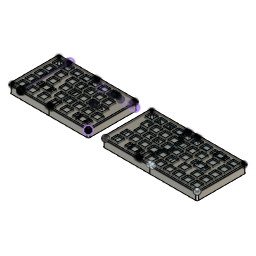
gKeyboard (Autodesk Fusion 360 design; units mm, degrees)
Autodesk Fusion 360 part; units mm, degrees
(part 1 of 3)
sketch "스케치2" plane through (0, 0, 0) normal (0, 0, 1) x (1, 0, 0) in component "leftKey"
  line L0 (0, 0) -> (-142.1125, 0)
  line L1 (-142.1125, 0) -> (-142.1125, 103.25)
  line L2 (-142.1125, 103.25) -> (0, 103.25)
  line L3 (0, 103.25) -> (0, 0)
  circle A0 centre (-3.1, 3.1) radius 1.55
  circle A1 centre (-139.0125, 3.1) radius 1.55
  line L4 (-137.2063, 20.525) -> (-123.2063, 20.525)
  line L5 (-123.2063, 20.525) -> (-123.2063, 6.525)
  line L6 (-123.2063, 6.525) -> (-137.2063, 6.525)
  line L7 (-137.2063, 6.525) -> (-137.2063, 20.525)
  line L8 (-99.3938, 6.525) -> (-113.3938, 6.525)
  line L9 (-113.3938, 6.525) -> (-113.3938, 20.525)
  line L10 (-113.3938, 20.525) -> (-99.3938, 20.525)
  line L11 (-99.3938, 20.525) -> (-99.3938, 6.525)
  line L12 (-75.5813, 6.525) -> (-89.5813, 6.525)
  line L13 (-89.5813, 6.525) -> (-89.5813, 20.525)
  line L14 (-89.5813, 20.525) -> (-75.5813, 20.525)
  line L15 (-75.5813, 20.525) -> (-75.5813, 6.525)
  line L16 (-51.7688, 6.525) -> (-65.7688, 6.525)
  line L17 (-65.7688, 6.525) -> (-65.7688, 20.525)
  line L18 (-65.7688, 20.525) -> (-51.7688, 20.525)
  line L19 (-51.7688, 20.525) -> (-51.7688, 6.525)
  line L20 (-82.725, 25.575) -> (-96.725, 25.575)
  line L21 (-96.725, 39.575) -> (-82.725, 39.575)
  line L22 (-96.725, 25.575) -> (-96.725, 39.575)
  line L23 (-82.725, 39.575) -> (-82.725, 25.575)
  line L24 (-63.675, 25.575) -> (-77.675, 25.575)
  line L25 (-77.675, 25.575) -> (-77.675, 39.575)
  line L26 (-63.675, 39.575) -> (-63.675, 25.575)
  line L27 (-77.675, 39.575) -> (-63.675, 39.575)
  line L28 (-44.625, 25.575) -> (-58.625, 25.575)
  line L29 (-58.625, 25.575) -> (-58.625, 39.575)
  line L30 (-44.625, 39.575) -> (-44.625, 25.575)
  line L31 (-58.625, 39.575) -> (-44.625, 39.575)
  line L32 (-25.575, 25.575) -> (-39.575, 25.575)
  line L33 (-39.575, 25.575) -> (-39.575, 39.575)
  line L34 (-25.575, 39.575) -> (-25.575, 25.575)
  line L35 (-39.575, 39.575) -> (-25.575, 39.575)
  line L36 (-6.525, 25.575) -> (-20.525, 25.575)
  line L37 (-20.525, 25.575) -> (-20.525, 39.575)
  line L38 (-6.525, 39.575) -> (-6.525, 25.575)
  line L39 (-20.525, 39.575) -> (-6.525, 39.575)
  line L40 (-132.4438, 58.625) -> (-118.4438, 58.625)
  line L41 (-132.4438, 44.625) -> (-132.4438, 58.625)
  line L42 (-118.4438, 58.625) -> (-118.4438, 44.625)
  line L43 (-118.4438, 44.625) -> (-132.4438, 44.625)
  line L44 (-106.25, 58.625) -> (-92.25, 58.625)
  line L45 (-106.25, 44.625) -> (-106.25, 58.625)
  line L46 (-92.25, 58.625) -> (-92.25, 44.625)
  line L47 (-92.25, 44.625) -> (-106.25, 44.625)
  line L48 (-73.2, 44.625) -> (-87.2, 44.625)
  line L49 (-87.2, 44.625) -> (-87.2, 58.625)
  line L50 (-73.2, 58.625) -> (-73.2, 44.625)
  line L51 (-87.2, 58.625) -> (-73.2, 58.625)
  line L52 (-54.15, 44.625) -> (-68.15, 44.625)
  line L53 (-68.15, 44.625) -> (-68.15, 58.625)
  line L54 (-54.15, 58.625) -> (-54.15, 44.625)
  line L55 (-68.15, 58.625) -> (-54.15, 58.625)
  line L56 (-35.1, 44.625) -> (-49.1, 44.625)
  line L57 (-49.1, 44.625) -> (-49.1, 58.625)
  line L58 (-35.1, 58.625) -> (-35.1, 44.625)
  line L59 (-49.1, 58.625) -> (-35.1, 58.625)
  line L60 (-16.05, 44.625) -> (-30.05, 44.625)
  line L61 (-30.05, 44.625) -> (-30.05, 58.625)
  line L62 (-16.05, 58.625) -> (-16.05, 44.625)
  line L63 (-30.05, 58.625) -> (-16.05, 58.625)
  line L64 (-120.825, 63.675) -> (-134.825, 63.675)
  line L65 (-134.825, 63.675) -> (-134.825, 77.675)
  line L66 (-120.825, 77.675) -> (-120.825, 63.675)
  line L67 (-134.825, 77.675) -> (-120.825, 77.675)
  line L68 (-111.0125, 63.675) -> (-111.0125, 77.675)
  line L69 (-97.0125, 63.675) -> (-111.0125, 63.675)
  line L70 (-97.0125, 77.675) -> (-97.0125, 63.675)
  line L71 (-111.0125, 77.675) -> (-97.0125, 77.675)
  line L72 (-91.9625, 77.675) -> (-77.9625, 77.675)
  line L73 (-77.9625, 77.675) -> (-77.9625, 63.675)
  line L74 (-77.9625, 63.675) -> (-91.9625, 63.675)
  line L75 (-91.9625, 63.675) -> (-91.9625, 77.675)
  line L76 (-72.9125, 77.675) -> (-58.9125, 77.675)
  line L77 (-58.9125, 77.675) -> (-58.9125, 63.675)
  line L78 (-58.9125, 63.675) -> (-72.9125, 63.675)
  line L79 (-72.9125, 63.675) -> (-72.9125, 77.675)
  line L80 (-53.8625, 77.675) -> (-39.8625, 77.675)
  line L81 (-39.8625, 77.675) -> (-39.8625, 63.675)
  line L82 (-39.8625, 63.675) -> (-53.8625, 63.675)
  line L83 (-53.8625, 63.675) -> (-53.8625, 77.675)
  line L84 (-34.8125, 77.675) -> (-20.8125, 77.675)
  line L85 (-20.8125, 77.675) -> (-20.8125, 63.675)
  line L86 (-20.8125, 63.675) -> (-34.8125, 63.675)
  line L87 (-34.8125, 63.675) -> (-34.8125, 77.675)
  line L88 (-125.5875, 82.725) -> (-139.5875, 82.725)
  line L89 (-139.5875, 82.725) -> (-139.5875, 96.725)
  line L90 (-125.5875, 96.725) -> (-125.5875, 82.725)
  line L91 (-139.5875, 96.725) -> (-125.5875, 96.725)
  line L92 (-106.5375, 96.725) -> (-106.5375, 82.725)
  line L93 (-106.5375, 82.725) -> (-120.5375, 82.725)
  line L94 (-120.5375, 82.725) -> (-120.5375, 96.725)
  line L95 (-120.5375, 96.725) -> (-106.5375, 96.725)
  line L96 (-87.4875, 96.725) -> (-87.4875, 82.725)
  line L97 (-87.4875, 82.725) -> (-101.4875, 82.725)
  line L98 (-101.4875, 82.725) -> (-101.4875, 96.725)
  line L99 (-101.4875, 96.725) -> (-87.4875, 96.725)
  line L100 (-68.4375, 96.725) -> (-68.4375, 82.725)
  line L101 (-68.4375, 82.725) -> (-82.4375, 82.725)
  line L102 (-82.4375, 82.725) -> (-82.4375, 96.725)
  line L103 (-82.4375, 96.725) -> (-68.4375, 96.725)
  line L104 (-49.3875, 96.725) -> (-49.3875, 82.725)
  line L105 (-49.3875, 82.725) -> (-63.3875, 82.725)
  line L106 (-63.3875, 82.725) -> (-63.3875, 96.725)
  line L107 (-63.3875, 96.725) -> (-49.3875, 96.725)
  line L108 (-30.3375, 96.725) -> (-30.3375, 82.725)
  line L109 (-30.3375, 82.725) -> (-44.3375, 82.725)
  line L110 (-44.3375, 82.725) -> (-44.3375, 96.725)
  line L111 (-44.3375, 96.725) -> (-30.3375, 96.725)
  circle A2 centre (-139.0125, 100.15) radius 1.55
  circle A3 centre (-3.1, 100.15) radius 1.55
  line L112 (-18.4313, 14.625) -> (-16.9313, 14.625)
  line L113 (-33.9313, 12.425) -> (-33.9313, 7.925)
  line L114 (-32.4313, 12.425) -> (-33.9313, 12.425)
  line L115 (-33.9313, 7.925) -> (-40.7313, 7.925)
  line L116 (-16.9313, 19.125) -> (-10.1313, 19.125)
  line L117 (-16.9313, 14.625) -> (-16.9313, 19.125)
  line L118 (-18.4313, 6.525) -> (-32.4312, 6.525)
  line L119 (-32.4312, 20.525) -> (-18.4312, 20.525)
  line L120 (-10.1313, 7.925) -> (-16.9313, 7.925)
  line L121 (-16.9313, 12.425) -> (-18.4313, 12.425)
  line L122 (-32.4313, 14.625) -> (-32.4312, 20.525)
  line L123 (-40.7313, 19.125) -> (-33.9313, 19.125)
  line L124 (-33.9313, 19.125) -> (-33.9313, 14.625)
  line L125 (-18.4313, 12.425) -> (-18.4313, 6.525)
  line L126 (-16.9313, 7.925) -> (-16.9313, 12.425)
  line L127 (-18.4312, 20.525) -> (-18.4313, 14.625)
  line L128 (-32.4312, 6.525) -> (-32.4313, 12.425)
  line L129 (-10.1313, 19.125) -> (-10.1313, 7.925)
  line L130 (-33.9313, 14.625) -> (-32.4313, 14.625)
  line L131 (-40.7313, 7.925) -> (-40.7313, 19.125)
  line L132 (-113.6813, 25.575) -> (-127.6813, 25.575)
  line L133 (-127.6813, 39.575) -> (-113.6813, 39.575)
  line L134 (-129.1813, 26.975) -> (-135.9813, 26.975)
  line L135 (-129.1813, 33.675) -> (-127.6813, 33.675)
  line L136 (-113.6813, 39.575) -> (-113.6813, 33.675)
  line L137 (-112.1813, 26.975) -> (-112.1813, 31.475)
  line L138 (-112.1812, 38.175) -> (-105.3812, 38.175)
  line L139 (-129.1813, 38.175) -> (-129.1813, 33.675)
  line L140 (-113.6813, 33.675) -> (-112.1813, 33.675)
  line L141 (-127.6813, 31.475) -> (-129.1813, 31.475)
  line L142 (-135.9813, 26.975) -> (-135.9813, 38.175)
  line L143 (-105.3812, 26.975) -> (-112.1813, 26.975)
  line L144 (-112.1813, 33.675) -> (-112.1812, 38.175)
  line L145 (-135.9813, 38.175) -> (-129.1813, 38.175)
  line L146 (-112.1813, 31.475) -> (-113.6813, 31.475)
  line L147 (-127.6813, 25.575) -> (-127.6813, 31.475)
  line L148 (-129.1813, 31.475) -> (-129.1813, 26.975)
  line L149 (-105.3812, 38.175) -> (-105.3812, 26.975)
  line L150 (-113.6813, 31.475) -> (-113.6813, 25.575)
  line L151 (-127.6813, 33.675) -> (-127.6813, 39.575)
  line L152 (-82.5813, 103.25) -> (-82.5813, 0)
  circle A4 centre (-79.4813, 3.1) radius 1.55
  circle A5 centre (-85.6813, 3.1) radius 1.55
  circle A6 centre (-85.6813, 100.15) radius 1.55
  circle A7 centre (-79.4813, 100.15) radius 1.55
  point P0 (-195, 0)
  dimension "d6" = 3.1
  dimension "d8" = 3.1
  dimension "d9" = 3.1
  dimension "d12" = 3.1
  dimension "d14" = 3.1
  dimension "d15" = 3.1
  dimension "d16" = 142.1125
  dimension "d17" = 103.25
  dimension "d18" = 14
  dimension "d19" = 14
  dimension "d21" = 4.9063
  dimension "d22" = 6.525
  dimension "d25" = 23.8125
  dimension "d26" = 0
  dimension "d32" = 14
  dimension "d33" = 14
  dimension "d37" = 19.05
  dimension "d38" = 0
  dimension "d39" = 14
  dimension "d40" = 14
  dimension "d41" = 9.6688
  dimension "d43" = 14
  dimension "d44" = 14
  dimension "d45" = 12.1938
  dimension "d48" = 19.05
  dimension "d49" = 0
  dimension "d50" = 14
  dimension "d51" = 14
  dimension "d52" = 7.2875
  dimension "d53" = 19.05
  dimension "d54" = 14
  dimension "d55" = 14
  dimension "d56" = 9.8125
  dimension "d59" = 19.05
  dimension "d60" = 0
  dimension "d61" = 14
  dimension "d62" = 14
  dimension "d64" = 2.525
  dimension "d68" = 19.05
  dimension "d69" = 0
  dimension "d70" = 19.05
  dimension "d71" = 3.1
  dimension "d73" = 3.1
  dimension "d74" = 3.1
  dimension "d82" = 14
  dimension "d83" = 14
  dimension "d84" = 6.8
  dimension "d85" = 11.2
  dimension "d86" = 1.5
  dimension "d87" = 4.5
  dimension "d88" = 5.9
  dimension "d89" = 19.3375
  dimension "d90" = 14
  dimension "d91" = 14
  dimension "d92" = 6.8
  dimension "d93" = 11.2
  dimension "d94" = 1.5
  dimension "d95" = 4.5
  dimension "d96" = 5.9
  dimension "d97" = 19.05
  dimension "d98" = 14.4313
  dimension "d99" = 19.05
  dimension "d100" = 16.9563
  dimension "d196" = 82.5813
  dimension "d197" = 3.1
  dimension "d198" = 3.1
  dimension "d199" = 3.1
  dimension "d200" = 3.1
  dimension "d201" = 3.1
  dimension "d202" = 3.1
  dimension "d203" = 3.1
  dimension "d204" = 3.1
  constraint horizontal L0
  constraint vertical L1
  constraint horizontal L2
  constraint vertical L3
  constraint coincident L0.start L3.end
  constraint horizontal L4
  constraint vertical L5
  constraint horizontal L6
  constraint vertical L7
  constraint horizontal L21
  constraint vertical L23
  constraint horizontal L20
  constraint vertical L22
  constraint horizontal L40
  constraint vertical L42
  constraint horizontal L43
  constraint vertical L41
  constraint horizontal L44
  constraint vertical L46
  constraint horizontal L47
  constraint vertical L45
  constraint horizontal L40.end L44.start
  constraint horizontal L67
  constraint vertical L66
  constraint horizontal L64
  constraint vertical L65
  constraint horizontal L71
  constraint vertical L70
  constraint horizontal L69
  constraint vertical L68
  constraint horizontal L66.start L68.end
  constraint horizontal L91
  constraint vertical L90
  constraint horizontal L88
  constraint vertical L89
  constraint vertical A0.centre A3.centre
  constraint horizontal L119
  constraint vertical L127
  constraint horizontal L118
  constraint vertical L128
  constraint horizontal L123
  constraint vertical L124
  constraint horizontal L115
  constraint vertical L131
  constraint horizontal L130
  constraint horizontal L121
  constraint horizontal L116
  constraint vertical L129
  constraint horizontal L120
  constraint vertical L126
  constraint collinear L113 L124
  constraint coincident L114.start L121
  constraint collinear L122 L128
  constraint coincident L112.start L130
  constraint collinear L125 L127
  constraint collinear L117 L126
  constraint collinear L114 L121
  constraint collinear L112 L130
  constraint equal L116 L123
  constraint equal L129 L131
  constraint equal L117 L124
  constraint equal L112 L130
  constraint equal L113 L124
  constraint horizontal L18.end L119.start
  constraint horizontal L133
  constraint vertical L136
  constraint horizontal L132
  constraint vertical L147
  constraint horizontal L145
  constraint vertical L139
  constraint horizontal L134
  constraint vertical L142
  constraint horizontal L135
  constraint horizontal L146
  constraint horizontal L138
  constraint vertical L149
  constraint horizontal L143
  constraint vertical L137
  constraint collinear L139 L148
  constraint coincident L141.start L146
  constraint collinear L147 L151
  constraint coincident L136.end L135
  constraint collinear L136 L150
  constraint collinear L137 L144
  constraint collinear L141 L146
  constraint collinear L135 L140
  constraint equal L138 L145
  constraint equal L142 L149
  constraint equal L139 L144
  constraint equal L135 L140
  constraint equal L139 L148
  constraint horizontal L21.start L133.end
  constraint vertical A1.centre A2.centre
  constraint horizontal A2.centre A3.centre
  constraint coincident L2 L152.start
  constraint coincident L0 L152.end
  constraint perpendicular L0 L152
  constraint horizontal A0.centre A4.centre
  constraint horizontal A0.centre A5.centre
  constraint horizontal A3.centre A7.centre
  constraint horizontal A7.centre A6.centre
  measures "d6" diameter of A0
  measures "d8" horizontal distance of L0.start A0.centre
  measures "d9" vertical distance of L0.start A0.centre
  measures "d12" diameter of A1
  measures "d14" vertical distance of L0.end A1.centre
  measures "d15" horizontal distance of L0.end A1.centre
  measures "d16" distance of L0.start L0.end
  measures "d17" distance of L0.start L2.end
  measures "d18" distance of L4.start L4.end
  measures "d19" distance of L4.start L6.end
  measures "d21" horizontal distance of L0.end L6.end
  measures "d22" vertical distance of L0.end L6.end
  measures "d32" distance of L21.end L21.start
  measures "d33" distance of L20.end L21.start
  measures "d39" distance of L40.end L40.start
  measures "d40" distance of L41.start L40.start
  measures "d41" distance of L1 L41.start
  measures "d43" distance of L44.end L44.start
  measures "d44" distance of L45.start L44.start
  measures "d45" distance of L42.end L45.start
  measures "d50" distance of L66.start L65.end
  measures "d51" distance of L64.end L65.end
  measures "d52" distance of L1 L64.end
  measures "d53" vertical distance of L41.start L64.end
  measures "d54" distance of L70.start L68.end
  measures "d55" distance of L68.end L68.start
  measures "d56" distance of L64.start L68.start
  measures "d61" distance of L90.start L89.end
  measures "d62" distance of L89.end L88.end
  measures "d64" distance of L1 L88.end
  measures "d70" vertical distance of L64.end L88.end
  measures "d71" diameter of A2
  measures "d73" vertical distance of L1.end A2.centre
  measures "d74" diameter of A3
  measures "d82" distance of L119.start L119.end
  measures "d83" distance of L119.start L118.end
  measures "d84" distance of L123.start L123.end
  measures "d85" distance of L123.start L115.end
  measures "d86" distance of L122.start L124.end
  measures "d87" distance of L123.end L124.end
  measures "d88" distance of L122.start L119.start
  measures "d89" distance of L16.start L118.end
  measures "d90" distance of L133.end L133.start
  measures "d91" distance of L132.end L133.start
  measures "d92" distance of L139.start L142.end
  measures "d93" distance of L134.end L142.end
  measures "d94" distance of L135.end L135.start
  measures "d95" distance of L139.start L135.start
  measures "d96" distance of L135.end L133.start
  measures "d97" vertical distance of L6.end L132.end
  measures "d98" distance of L1 L132.end
  measures "d99" vertical distance of L41.start L132.end
  measures "d100" distance of L20.end L132.start
  measures "d196" distance of L0.start L152.end
  measures "d197" diameter of A4
  measures "d198" distance of L152 A4.centre
  measures "d199" diameter of A5
  measures "d200" distance of L152 A5.centre
  measures "d201" diameter of A7
  measures "d202" diameter of A6
  measures "d203" distance of L152 A7.centre
  measures "d204" distance of L152 A6.centre
extrude "돌출1" add sketch "스케치2" along normal blind 3 contours L0 L2 L3 L12 L14 L15 L48 L50 L51 L72 L73 L74 L152 | L0 L1 L2 L12 L13 L14 L48 L49 L51 L72 L74 L75 L152 makes body 1 in component "leftKey"
sketch "스케치3" plane through (0, 0, 3) normal (0, 0, 1) x (-1, 0, 0) in component "leftKey"
  circle A0 centre (139.0125, -100.15) radius 3
  circle A1 centre (3.1, -100.15) radius 3
  circle A2 centre (3.1, -3.1) radius 3
  circle A3 centre (139.0125, -3.1) radius 3
  circle A4 centre (79.4813, -3.1) radius 1.55
  circle A5 centre (85.6813, -3.1) radius 1.55
  circle A6 centre (79.4813, -100.15) radius 1.55
  circle A7 centre (85.6813, -100.15) radius 1.55
  circle A8 centre (79.4813, -100.15) radius 3
  circle A9 centre (85.6813, -100.15) radius 3
  circle A10 centre (79.4813, -3.1) radius 3
  circle A11 centre (85.6813, -3.1) radius 3
  point P0 (139.0125, -3.1)
  point P1 (3.1, -3.1)
  point P2 (139.0125, -100.15)
  point P3 (3.1, -100.15)
  point P4 (79.4813, -3.1)
  dimension "d103" = 6
  dimension "d104" = 6
  dimension "d105" = 6
  dimension "d106" = 6
  dimension "d205" = 6
  dimension "d206" = 6
  dimension "d207" = 6
  dimension "d208" = 6
  constraint coincident P2 A0.centre
  constraint coincident P3 A1.centre
  constraint coincident P1 A2.centre
  constraint coincident P0 A3.centre
  constraint concentric A6 A8
  constraint concentric A7 A9
  constraint concentric A4 A10
  constraint concentric A5 A11
  measures "d103" diameter of A0
  measures "d104" diameter of A1
  measures "d105" diameter of A2
  measures "d106" diameter of A3
  measures "d205" diameter of A8
  measures "d206" diameter of A9
  measures "d207" diameter of A10
  measures "d208" diameter of A11
extrude "돌출2" cut sketch "스케치3" against normal blind 1.75 bodies 1 in component "leftKey"
fillet "모깎기3" radius 3.1 2 edges at (0, 0, 1.5) (0, 103.25, 1.5) on bodies 1 in component "leftKey"
sketch "스케치1" plane through (0, 0, 0) normal (0, 0, 1) x (1, 0, 0) in component "sideKey"
  line L0 (-142.1125, 0) -> (-142.1125, 103.25)
  line L1 (-142.1125, 0) -> (-165.1625, 0)
  line L2 (-165.1625, 0) -> (-165.1625, 103.25)
  line L3 (-165.1625, 103.25) -> (-142.1125, 103.25)
  line L4 (-142.1125, 103.25) -> (-142.1125, 0)
  line L5 (-144.6375, 20.525) -> (-158.6375, 20.525)
  line L6 (-158.6375, 20.525) -> (-158.6375, 6.525)
  line L7 (-158.6375, 6.525) -> (-144.6375, 6.525)
  line L8 (-144.6375, 6.525) -> (-144.6375, 20.525)
  line L9 (-158.6375, 39.575) -> (-158.6375, 25.575)
  line L10 (-158.6375, 25.575) -> (-144.6375, 25.575)
  line L11 (-144.6375, 25.575) -> (-144.6375, 39.575)
  line L12 (-144.6375, 39.575) -> (-158.6375, 39.575)
  line L13 (-158.6375, 58.625) -> (-158.6375, 44.625)
  line L14 (-158.6375, 44.625) -> (-144.6375, 44.625)
  line L15 (-144.6375, 44.625) -> (-144.6375, 58.625)
  line L16 (-144.6375, 58.625) -> (-158.6375, 58.625)
  line L17 (-158.6375, 77.675) -> (-158.6375, 63.675)
  line L18 (-158.6375, 63.675) -> (-144.6375, 63.675)
  line L19 (-144.6375, 63.675) -> (-144.6375, 77.675)
  line L20 (-144.6375, 77.675) -> (-158.6375, 77.675)
  line L21 (-158.6375, 96.725) -> (-158.6375, 82.725)
  line L22 (-158.6375, 82.725) -> (-144.6375, 82.725)
  line L23 (-144.6375, 82.725) -> (-144.6375, 96.725)
  line L24 (-144.6375, 96.725) -> (-158.6375, 96.725)
  circle A0 centre (-145.2125, 3.1) radius 1.55
  circle A1 centre (-162.0625, 3.1) radius 1.55
  circle A2 centre (-145.2125, 100.15) radius 1.55
  circle A3 centre (-162.0625, 100.15) radius 1.55
  dimension "d109" = 23.05
  dimension "d110" = 103.25
  dimension "d111" = 14
  dimension "d112" = 14
  dimension "d113" = 6.525
  dimension "d114" = 2.525
  dimension "d117" = 0
  dimension "d118" = 19.05
  dimension "d119" = 3.1
  dimension "d120" = 3.1
  dimension "d121" = 3.1
  dimension "d122" = 3.1
  dimension "d123" = 3.1
  dimension "d124" = 3.1
  dimension "d125" = 3.1
  dimension "d126" = 3.1
  constraint horizontal L1
  constraint vertical L2
  constraint horizontal L3
  constraint vertical L4
  constraint coincident L0.start L1.start
  constraint horizontal L5
  constraint vertical L6
  constraint horizontal L7
  constraint vertical L8
  constraint horizontal A0.centre A1.centre
  constraint vertical A0.centre A2.centre
  constraint horizontal A2.centre A3.centre
  constraint vertical A1.centre A3.centre
  measures "d109" distance of L0.start L1.end
  measures "d110" distance of L1.end L2.end
  measures "d111" distance of L5.start L5.end
  measures "d112" distance of L5.start L7.end
  measures "d113" vertical distance of L0.start L7.end
  measures "d114" horizontal distance of L0.start L7.end
  measures "d119" diameter of A0
  measures "d120" horizontal distance of L0.start A0.centre
  measures "d121" vertical distance of L0.start A0.centre
  measures "d122" diameter of A1
  measures "d123" horizontal distance of L1.end A1.centre
  measures "d124" diameter of A2
  measures "d125" vertical distance of L0.end A2.centre
  measures "d126" diameter of A3
extrude "돌출1'" add sketch "스케치1" along normal blind 3 separate body makes body 2 in component "sideKey"
sketch "스케치2 (2)" plane through (0, 0, 3) normal (0, 0, 1) x (-1, 0, 0) in component "sideKey"
  circle A0 centre (162.0625, -100.15) radius 1.55
  circle A1 centre (145.2125, -100.15) radius 1.55
  circle A2 centre (162.0625, -3.1) radius 1.55
  circle A3 centre (145.2125, -3.1) radius 1.55
  circle A4 centre (145.2125, -3.1) radius 3
  circle A5 centre (162.0625, -3.1) radius 3
  circle A6 centre (145.2125, -100.15) radius 3
  circle A7 centre (162.0625, -100.15) radius 3
  dimension "d129" = 6
  dimension "d130" = 6
  dimension "d131" = 6
  dimension "d132" = 6
  constraint concentric A3 A4
  constraint concentric A2 A5
  constraint concentric A1 A6
  constraint concentric A0 A7
  measures "d129" diameter of A4
  measures "d130" diameter of A5
  measures "d131" diameter of A6
  measures "d132" diameter of A7
extrude "돌출2'" cut sketch "스케치2 (2)" against normal blind 1.75 bodies 2 in component "sideKey"
sketch "스케치1 (2)" plane through (0, 0, 0) normal (0, 0, 1) x (1, 0, 0) in component "leftBody1"
  line L0 (0, 0) -> (-142.1125, 0)
  line L1 (-142.1125, 0) -> (-165.1625, 0)
  line L2 (-165.1625, 0) -> (-165.1625, 103.25)
  line L3 (-165.1625, 103.25) -> (-142.1125, 103.25)
  line L4 (-142.1125, 103.25) -> (0, 103.25)
  line L5 (0, 103.25) -> (0, 0)
  circle A0 centre (-162.0625, 100.15) radius 1.55
  circle A1 centre (-145.2125, 100.15) radius 1.55
  circle A2 centre (-145.2125, 3.1) radius 1.55
  circle A3 centre (-162.0625, 3.1) radius 1.55
  circle A4 centre (-139.0125, 100.15) radius 1.55
  circle A5 centre (-139.0125, 3.1) radius 1.55
  circle A6 centre (-3.1, 3.1) radius 1.55
  circle A7 centre (-3.1, 100.15) radius 1.55
  line L6 (0, 0) -> (-82.5813, 0)
  line L7 (-82.5813, 0) -> (-82.5813, 103.25)
  line L8 (-82.5813, 103.25) -> (0, 103.25)
  line L9 (0, 103.25) -> (0, 0)
  circle A8 centre (-3.1, 3.1) radius 1.5
  circle A9 centre (-3.1, 100.15) radius 1.5
  circle A10 centre (-79.5813, 3.1) radius 1.5
  circle A11 centre (-79.5813, 100.15) radius 1.5
  arc A12 (-77.1543, 2.5) -> (-82.0082, 2.5) centre (-79.5813, 3.1) ccw
  line L10 (-82.5813, 2.5) -> (-82.0082, 2.5)
  arc A13 (-2.5, 5.5269) -> (-5.5269, 2.5) centre (-3.1, 3.1) ccw
  line L11 (-77.1543, 2.5) -> (-5.5269, 2.5)
  line L12 (-4.5292, 2.5) -> (-4.4748, 2.5)
  line L13 (-1.7252, 2.5) -> (-1.6708, 2.5)
  line L14 (-2.5, 1.6708) -> (-2.5, 1.7252)
  line L15 (-2.5, 4.4748) -> (-2.5, 4.5292)
  arc A14 (-82.0082, 100.75) -> (-77.1543, 100.75) centre (-79.5813, 100.15) ccw
  line L16 (-82.5813, 100.75) -> (-82.0082, 100.75)
  arc A15 (-5.5269, 100.75) -> (-2.5, 97.7231) centre (-3.1, 100.15) ccw
  line L17 (-2.5, 101.5248) -> (-2.5, 101.5792)
  line L18 (-1.7252, 100.75) -> (-1.6708, 100.75)
  line L19 (-77.1543, 100.75) -> (-5.5269, 100.75)
  line L20 (-4.5292, 100.75) -> (-4.4748, 100.75)
  line L21 (-2.5, 5.5269) -> (-2.5, 97.7231)
  line L22 (-2.5, 98.7208) -> (-2.5, 98.7752)
  point P0 (-3.1, 3.1)
  point P1 (-3.1, 100.15)
  point P2 (-139.0125, 3.1)
  point P3 (-139.0125, 100.15)
  point P4 (-79.5813, 100.15)
  dimension "d136" = 82.5813
  dimension "d137" = 3
  dimension "d138" = 3
  dimension "d139" = 3
  dimension "d140" = 3
  dimension "d141" = 3
  dimension "d142" = 5
  dimension "d145" = 5
  dimension "d146" = 5
  dimension "d147" = 5
  dimension "d149" = 2.5
  dimension "d151" = 2.5
  dimension "d152" = 2.5
  dimension "d153" = 2.5
  constraint horizontal L6
  constraint vertical L7
  constraint horizontal L8
  constraint vertical L9
  constraint coincident L4 L7.end
  constraint coincident L0.start L5.end
  constraint concentric A6 A8
  constraint coincident P1 A7.centre
  constraint horizontal P0 A10.centre
  constraint vertical A10.centre P4
  constraint horizontal P1 P4
  constraint coincident P4 A11.centre
  constraint concentric A7 A15
  constraint concentric A8 A13
  constraint concentric A10 A12
  constraint coincident L7 L10.start
  constraint perpendicular L5 L10
  constraint coincident A12.start L10
  constraint coincident A6 L12.start
  constraint collinear L11 L12
  constraint coincident A8 L12.end
  constraint coincident A8 L13.start
  constraint collinear L12 L13
  constraint perpendicular L4 L14
  constraint coincident A6 L15.end
  constraint collinear L14 L21
  constraint coincident A6 L13.end
  constraint coincident A6 L14.start
  constraint coincident A8 L14.end
  constraint coincident A8 L15.start
  constraint collinear L14 L15
  constraint coincident L7 L16.start
  constraint perpendicular L5 L16
  constraint coincident A14.end L16
  constraint collinear L16 L19
  constraint coincident A7 L17.end
  constraint coincident A9 L20.end
  constraint collinear L18 L19
  constraint coincident A9 L17.start
  constraint collinear L17 L21
  constraint coincident A9 L18.start
  constraint coincident A9 L22.end
  constraint coincident A7 L18.end
  constraint coincident A7 L20.start
  constraint collinear L19 L20
  constraint coincident A7 L22.start
  constraint collinear L21 L22
  measures "d136" distance of L0.start L6.end
  measures "d137" diameter of A8
  measures "d138" diameter of A9
  measures "d139" diameter of A10
  measures "d140" horizontal distance of L6.end A10.centre
  measures "d141" diameter of A11
  measures "d142" diameter of A14
  measures "d145" diameter of A15
  measures "d146" diameter of A13
  measures "d147" diameter of A12
  measures "d149" distance of L6.end L10.start
  measures "d151" distance of L6 A13.end
  measures "d152" distance of L9 A13.start
  measures "d153" distance of L7.end L16.start
extrude "돌출1''" add sketch "스케치1 (2)" against normal blind 15 separate body contours L0 L4 L5 L6 L7 L8 L9 A12 L10 A13 L11 A14 L16 A15 L19 L21 | L7 A12 L10 A13 L11 A14 L16 A15 L19 L21 | A6 A8 L13 L15 | A6 A8 L12 L15 | A6 A8 L13 L14 | A6 A8 L12 L14 | A8 | A7 A9 L18 L22 | A7 A9 L17 L18 | A7 A9 L20 L22 | A7 A9 L17 L20 | A9 | A10 | A11 makes body 3 in component "leftBody1"
extrude "돌출2''" cut sketch "스케치1 (2)" against normal blind 13 contours L7 A12 L10 A13 L11 A14 L16 A15 L19 L21 bodies 3 in component "leftBody1"
extrude "돌출3" cut sketch "스케치1 (2)" against normal blind 10 contours A8 | A9 | A10 | A11 bodies 3 in component "leftBody1"
sketch "스케치1 (3)" plane through (0, 0, 0) normal (0, 0, 1) x (1, 0, 0) in component "leftBody2"
  line L0 (-142.1125, 0) -> (-165.1625, 0)
  line L1 (0, 0) -> (-142.1125, 0)
  line L2 (-165.1625, 0) -> (-165.1625, 103.25)
  line L3 (-165.1625, 103.25) -> (-142.1125, 103.25)
  line L4 (-142.1125, 103.25) -> (0, 103.25)
  circle A0 centre (-162.0625, 100.15) radius 1.55
  circle A1 centre (-162.0625, 3.1) radius 1.55
  circle A2 centre (-145.2125, 3.1) radius 1.55
  circle A3 centre (-139.0125, 3.1) radius 1.55
  circle A4 centre (-145.2125, 100.15) radius 1.55
  circle A5 centre (-139.0125, 100.15) radius 1.55
  line L5 (-82.5817, 103.25) -> (-165.163, 103.25)
  line L6 (-165.163, 103.25) -> (-165.163, 0)
  line L7 (-165.163, 0) -> (-82.5817, 0)
  line L8 (-82.5817, 0) -> (-82.5817, 103.25)
  circle A6 centre (-162.0625, 3.1) radius 1.5
  circle A7 centre (-145.2125, 3.1) radius 1.5
  circle A8 centre (-139.0125, 3.1) radius 1.5
  circle A9 centre (-162.0625, 100.15) radius 1.5
  circle A10 centre (-145.2125, 100.15) radius 1.5
  circle A11 centre (-139.0125, 100.15) radius 1.5
  circle A12 centre (-85.6817, 100.15) radius 1.5
  circle A13 centre (-85.6813, 3.1) radius 1.5
  arc A14 (-83.2543, 2.5) -> (-88.1082, 2.5) centre (-85.6813, 3.1) ccw
  line L9 (-82.5817, 2.5) -> (-83.2543, 2.5)
  arc A15 (-136.5856, 2.5) -> (-141.4394, 2.5) centre (-139.0125, 3.1) ccw
  line L10 (-88.1082, 2.5) -> (-136.5856, 2.5)
  arc A16 (-142.7856, 2.5) -> (-147.6394, 2.5) centre (-145.2125, 3.1) ccw
  line L11 (-141.4394, 2.5) -> (-142.7856, 2.5)
  arc A17 (-159.6356, 2.5) -> (-162.663, 5.5268) centre (-162.0625, 3.1) ccw
  line L12 (-162.663, 1.671) -> (-162.663, 1.7254)
  line L13 (-147.6394, 2.5) -> (-159.6356, 2.5)
  arc A18 (-162.663, 97.7232) -> (-159.6356, 100.75) centre (-162.0625, 100.15) ccw
  line L14 (-162.663, 5.5268) -> (-162.663, 97.7232)
  line L15 (-165.163, 100.75) -> (-165.1625, 100.75)
  line L16 (-159.6356, 100.75) -> (-147.6394, 100.75)
  arc A19 (-147.6394, 100.75) -> (-142.7856, 100.75) centre (-145.2125, 100.15) ccw
  arc A20 (-141.4394, 100.75) -> (-136.5856, 100.75) centre (-139.0125, 100.15) ccw
  line L17 (-142.7856, 100.75) -> (-141.4394, 100.75)
  arc A21 (-88.1087, 100.75) -> (-83.2548, 100.75) centre (-85.6817, 100.15) ccw
  line L18 (-136.5856, 100.75) -> (-88.1087, 100.75)
  line L19 (-83.2548, 100.75) -> (-82.5817, 100.75)
  point P0 (-139.0125, 100.15)
  point P1 (-145.2125, 100.15)
  point P2 (-162.0625, 100.15)
  point P3 (-82.5813, 0)
  point P4 (0, 103.25)
  dimension "d163" = 82.5813
  dimension "d164" = 103.25
  dimension "d165" = 3
  dimension "d166" = 3
  dimension "d167" = 3
  dimension "d168" = 3
  dimension "d169" = 3
  dimension "d170" = 3
  dimension "d171" = 3
  dimension "d172" = 3.1
  dimension "d173" = 3
  dimension "d174" = 3.1
  dimension "d175" = 5
  dimension "d176" = 5
  dimension "d177" = 5
  dimension "d178" = 5
  dimension "d179" = 5
  dimension "d180" = 5
  dimension "d181" = 5
  dimension "d182" = 5
  dimension "d183" = 2.5
  dimension "d185" = 2.5
  dimension "d186" = 2.5
  dimension "d187" = 2.5
  dimension "d188" = 82.5817
  dimension "d189" = 2.5
  constraint horizontal L5
  constraint vertical L6
  constraint horizontal L7
  constraint vertical L8
  constraint coincident L4 L5.start
  constraint concentric A1 A6
  constraint concentric A2 A7
  constraint concentric A3 A8
  constraint concentric A0 A9
  constraint coincident P1 A4.centre
  constraint coincident P0 A5.centre
  constraint horizontal P0 A12.centre
  constraint horizontal A3.centre A13.centre
  constraint concentric A13 A14
  constraint concentric A8 A15
  constraint concentric A2 A16
  constraint concentric A6 A17
  constraint coincident P2 A0.centre
  constraint concentric A4 A19
  constraint concentric A12 A21
  constraint coincident L8 L9.start
  constraint perpendicular L8 L9
  constraint perpendicular L3 L12
  constraint coincident L6 L15.start
  constraint coincident L8 L19.end
  constraint perpendicular L8 L15
  constraint coincident A14.end L9
  constraint collinear L9 L10
  constraint coincident A15.end L10
  constraint coincident A16.end L11
  constraint coincident A17.end L12
  constraint coincident A1 L12.start
  constraint coincident A6 L12.end
  constraint coincident L2 L15.end
  constraint collinear L16 L17
  constraint coincident A20.end L17
  constraint coincident A21.end L18
  constraint horizontal L18
  constraint horizontal L19
  constraint vertical L14
  constraint horizontal L13
  measures "d163" distance of L5.start L5.end
  measures "d164" distance of L5.end L6.end
  measures "d165" diameter of A6
  measures "d166" diameter of A7
  measures "d167" diameter of A8
  measures "d168" diameter of A9
  measures "d169" diameter of A10
  measures "d170" diameter of A11
  measures "d171" diameter of A12
  measures "d172" horizontal distance of L5.start A12.centre
  measures "d173" diameter of A13
  measures "d174" horizontal distance of A13.centre P3
  measures "d175" diameter of A14
  measures "d176" diameter of A15
  measures "d177" diameter of A16
  measures "d178" diameter of A17
  measures "d179" diameter of A18
  measures "d180" diameter of A19
  measures "d181" diameter of A20
  measures "d182" diameter of A21
  measures "d183" distance of L7.end L9.start
  measures "d185" distance of L5 L15
  measures "d186" distance of L6 L12
  measures "d187" distance of L5 L16
  measures "d188" distance of L5.start P4
  measures "d189" distance of L7 L13
extrude "돌출1'''" add sketch "스케치1 (3)" against normal blind 15 separate body contours L0 L1 L2 L3 L4 L5 L6 L7 L8 A14 L9 A15 L10 A16 L11 A17 L13 A18 L14 L16 A19 A20 L17 A21 L18 L19 | L8 A14 L9 A15 L10 A16 L11 A17 L13 A18 L14 L16 A19 A20 L17 A21 L18 L19 | A0 | A1 | A2 | A3 | A4 | A5 | A6 | A7 | A8 | A9 | A10 | A11 | A12 | A13 makes body 4 in component "leftBody2"
extrude "돌출2'''" cut sketch "스케치1 (3)" against normal blind 13 contours L8 A14 L9 A15 L10 A16 L11 A17 L13 A18 L14 L16 A19 A20 L17 A21 L18 L19 bodies 4 in component "leftBody2"
extrude "돌출3'" cut sketch "스케치1 (3)" against normal blind 10 contours A6 | A7 | A8 | A9 | A10 | A11 | A12 | A13 bodies 4 in component "leftBody2"
fillet "모깎기1" radius 3.1 2 edges at (-165.1625, 103.25, 1.5) (-165.1625, 0, 1.5) on bodies 2 in component "sideKey"
fillet "모깎기1'" radius 3.1 2 edges at (0, 103.25, -7.5) (0, 0, -7.5) on bodies 3 in component "leftBody1"
sketch "스케치2 (3)" plane through (0, 0, -13) normal (0, 0, 1) x (-1, 0, 0) in component "leftBody1"
  line L0 (77.1543, -100.75) -> (5.5269, -100.75)
  line L1 (20.5269, -85.75) -> (8.5269, -85.75)
  line L2 (8.5269, -85.75) -> (8.5269, -84.75)
  line L3 (8.5269, -84.75) -> (20.5269, -84.75)
  line L4 (20.5269, -84.75) -> (20.5269, -85.75)
  line L5 (53.5269, -65.15) -> (35.5269, -65.15)
  line L6 (35.5269, -65.15) -> (35.5269, -64.15)
  line L7 (35.5269, -64.15) -> (53.5269, -64.15)
  line L8 (53.5269, -64.15) -> (53.5269, -65.15)
  dimension "d223" = 12
  dimension "d224" = 1
  dimension "d225" = 15
  dimension "d226" = 3
  dimension "d227" = 18
  dimension "d228" = 1
  dimension "d229" = 30
  dimension "d230" = 35.6
  constraint horizontal L1
  constraint vertical L2
  constraint horizontal L3
  constraint vertical L4
  constraint horizontal L5
  constraint vertical L6
  constraint horizontal L7
  constraint vertical L8
  measures "d223" distance of L2.end L3.end
  measures "d224" distance of L1.start L3.end
  measures "d225" distance of L0 L1
  measures "d226" horizontal distance of L0.end L1.end
  measures "d227" distance of L5.start L5.end
  measures "d228" distance of L5.start L7.end
  measures "d229" horizontal distance of L0.end L6.end
  measures "d230" distance of L0 L5.end
extrude "돌출4" add sketch "스케치2 (3)" along normal blind 2 bodies 3 in component "leftBody1"
sketch "스케치3 (2)" plane through (-53.5269, 0, 0) normal (-1, 0, 0) x (0, -1, 0) in component "leftBody1"
  line L0 (-65.15, -11) -> (-64.15, -11)
  line L1 (-64.15, -11) -> (-64.15, -10.4348)
  line L2 (-64.8262, -10.1455) -> (-65.7214, -11)
  line L3 (-65.7214, -11) -> (-65.15, -11)
  arc A0 (-64.15, -10.4348) -> (-64.8262, -10.1455) centre (-64.55, -10.4348) ccw
  point P0 (-64.15, -9.5)
  dimension "d233" = 1.5
  dimension "d234" = 0.4
  constraint coincident L0.end L1.start
  constraint perpendicular L0 L1
  constraint coincident L0.start L3.end
  constraint perpendicular L1 L3
  constraint coincident P0 L2
  constraint coincident P0 L1
  constraint tangent L2 A0
  constraint tangent L1 A0
  measures "d233" distance of L0.end P0
  measures "d234" radius of A0
extrude "돌출5" add sketch "스케치3 (2)" against normal blind 18 bodies 3 in component "leftBody1"
sketch "스케치4" plane through (0, 103.25, 0) normal (0, 1, 0) x (-1, 0, 0) in component "leftBody1"
  line L0 (77.1543, -13) -> (5.5269, -13)
  line L1 (20.5269, -13) -> (8.5269, -13)
  line L2 (53.5269, -13) -> (35.5269, -13)
  circle A0 centre (12.5269, -10) radius 3.2
  line L3 (41.6269, -11.5) -> (47.4269, -11.5)
  arc A1 (47.4269, -11.5) -> (47.4269, -7.9) centre (47.4269, -9.7) ccw
  line L4 (47.4269, -7.9) -> (41.6269, -7.9)
  arc A2 (41.6269, -7.9) -> (41.6269, -11.5) centre (41.6269, -9.7) ccw
  line L5 (41.6269, -9.7) -> (47.4269, -9.7) construction
  line L6 (35.5269, -13) -> (53.5269, -13) construction
  line L7 (41.6269, -13.4) -> (47.4269, -13.4)
  arc A3 (47.4269, -13.4) -> (47.4269, -6) centre (47.4269, -9.7) ccw
  line L8 (47.4269, -6) -> (41.6269, -6)
  arc A4 (41.6269, -6) -> (41.6269, -13.4) centre (41.6269, -9.7) ccw
  line L9 (41.6269, -9.7) -> (47.4269, -9.7) construction
  dimension "d237" = 6.4
  dimension "d238" = 3
  dimension "d239" = 7
  dimension "d240" = 3.6
  dimension "d241" = 5.8
  dimension "d242" = 6.1
  dimension "d243" = 3.3
  dimension "d244" = 7.4
  constraint tangent L3 A1
  constraint tangent A1 L4
  constraint parallel L3 L4
  constraint tangent L4 A2
  constraint tangent L3 A2
  constraint horizontal L5
  constraint coincident L2.end L6.start
  constraint coincident L2.start L6.end
  constraint tangent L7 A3
  constraint tangent A3 L8
  constraint parallel L7 L8
  constraint tangent L8 A4
  constraint tangent L7 A4
  constraint coincident A1.centre L5.end
  constraint parallel L5 L9
  constraint coincident A2.centre L5.start
  measures "d237" diameter of A0
  measures "d238" distance of L0 A0.centre
  measures "d239" horizontal distance of L0.end A0.centre
  measures "d240" diameter of A1
  measures "d241" distance of A2.centre A1.centre
  measures "d242" horizontal distance of A2.centre L2.end
  measures "d243" distance of A2.centre L6
  measures "d244" diameter of A3
extrude "돌출6" cut sketch "스케치4" against normal blind 2.5 contours L0 L1 A0 | L3 A1 L4 A2 picked at (13.5671, -11.299) bodies 3 in component "leftBody1"
extrude "돌출7" cut sketch "스케치4" against normal blind 1.5 contours L0 L2 A3 L8 A4 bodies 3 in component "leftBody1"
sketch "스케치1 (4)" plane through (0, 0, 0) normal (0, 0, 1) x (1, 0, 0) in component "rightKey1"
  line L0 (50.8125, 44.625) -> (50.8125, 58.625)
  line L1 (64.8125, 58.625) -> (64.8125, 44.625)
  line L2 (30, 103.25) -> (30, 0)
  circle A0 centre (33.1, 3.1) radius 1.55
  line L3 (41.2875, 39.575) -> (55.2875, 39.575)
  line L4 (77.0062, 6.525) -> (77.0062, 12.425)
  line L5 (55.2875, 25.575) -> (41.2875, 25.575)
  line L6 (75.5062, 14.625) -> (77.0062, 14.625)
  line L7 (99.3063, 7.925) -> (92.5062, 7.925)
  line L8 (50.8125, 58.625) -> (64.8125, 58.625)
  line L9 (55.2875, 6.525) -> (41.2875, 6.525)
  line L10 (110.2, 103.25) -> (30, 103.25)
  line L11 (30, 0) -> (104.5156, 0)
  circle A1 centre (225.4, 3.1) radius 1.55
  line L12 (50.525, 82.725) -> (36.525, 82.725)
  line L13 (75.5062, 7.925) -> (68.7062, 7.925)
  line L14 (46.05, 63.675) -> (46.05, 77.675)
  line L15 (92.5062, 14.625) -> (92.5062, 19.125)
  line L16 (92.5062, 7.925) -> (92.5062, 12.425)
  line L17 (36.525, 96.725) -> (50.525, 96.725)
  line L18 (91.0062, 6.525) -> (77.0062, 6.525)
  line L19 (75.5062, 19.125) -> (75.5062, 14.625)
  line L20 (92.5062, 12.425) -> (91.0062, 12.425)
  line L21 (68.7062, 19.125) -> (75.5062, 19.125)
  line L22 (36.525, 82.725) -> (36.525, 96.725)
  line L23 (41.2875, 20.525) -> (55.2875, 20.525)
  line L24 (77.0062, 12.425) -> (75.5062, 12.425)
  line L25 (75.5062, 12.425) -> (75.5062, 7.925)
  line L26 (77.0062, 14.625) -> (77.0063, 20.525)
  line L27 (46.05, 77.675) -> (60.05, 77.675)
  line L28 (64.8125, 44.625) -> (50.8125, 44.625)
  line L29 (91.0063, 20.525) -> (91.0062, 14.625)
  line L30 (60.05, 63.675) -> (46.05, 63.675)
  line L31 (55.2875, 39.575) -> (55.2875, 25.575)
  line L32 (55.2875, 20.525) -> (55.2875, 6.525)
  line L33 (91.0062, 12.425) -> (91.0062, 6.525)
  circle A2 centre (33.1, 100.15) radius 1.55
  line L34 (99.3062, 19.125) -> (99.3063, 7.925)
  line L35 (77.0063, 20.525) -> (91.0063, 20.525)
  line L36 (92.5062, 19.125) -> (99.3062, 19.125)
  line L37 (41.2875, 25.575) -> (41.2875, 39.575)
  line L38 (68.7062, 7.925) -> (68.7062, 19.125)
  line L39 (41.2875, 6.525) -> (41.2875, 20.525)
  line L40 (60.05, 77.675) -> (60.05, 63.675)
  line L41 (50.525, 96.725) -> (50.525, 82.725)
  line L42 (91.0062, 14.625) -> (92.5062, 14.625)
  line L43 (114.9625, 23.05) -> (104.5156, 23.05)
  line L44 (114.9625, 42.1) -> (114.9625, 23.05)
  line L45 (124.4875, 42.1) -> (124.4875, 61.15)
  line L46 (119.725, 61.15) -> (124.4875, 61.15)
  line L47 (119.725, 80.2) -> (119.725, 61.15)
  line L48 (110.2, 80.2) -> (119.725, 80.2)
  line L49 (110.2, 80.2) -> (110.2, 103.25)
  line L50 (104.5156, 23.05) -> (104.5156, 0)
  line L51 (114.9625, 42.1) -> (124.4875, 42.1)
  line L52 (69.575, 82.725) -> (55.575, 82.725)
  line L53 (69.575, 96.725) -> (69.575, 82.725)
  line L54 (55.575, 96.725) -> (69.575, 96.725)
  line L55 (55.575, 82.725) -> (55.575, 96.725)
  line L56 (88.625, 82.725) -> (74.625, 82.725)
  line L57 (88.625, 96.725) -> (88.625, 82.725)
  line L58 (74.625, 96.725) -> (88.625, 96.725)
  line L59 (74.625, 82.725) -> (74.625, 96.725)
  line L60 (107.675, 82.725) -> (93.675, 82.725)
  line L61 (107.675, 96.725) -> (107.675, 82.725)
  line L62 (93.675, 96.725) -> (107.675, 96.725)
  line L63 (93.675, 82.725) -> (93.675, 96.725)
  line L64 (79.1, 63.675) -> (65.1, 63.675)
  line L65 (65.1, 63.675) -> (65.1, 77.675)
  line L66 (65.1, 77.675) -> (79.1, 77.675)
  line L67 (79.1, 77.675) -> (79.1, 63.675)
  line L68 (98.15, 63.675) -> (84.15, 63.675)
  line L69 (84.15, 63.675) -> (84.15, 77.675)
  line L70 (84.15, 77.675) -> (98.15, 77.675)
  line L71 (98.15, 77.675) -> (98.15, 63.675)
  line L72 (117.2, 63.675) -> (103.2, 63.675)
  line L73 (103.2, 63.675) -> (103.2, 77.675)
  line L74 (103.2, 77.675) -> (117.2, 77.675)
  line L75 (117.2, 77.675) -> (117.2, 63.675)
  line L76 (69.8625, 44.625) -> (69.8625, 58.625)
  line L77 (69.8625, 58.625) -> (83.8625, 58.625)
  line L78 (83.8625, 58.625) -> (83.8625, 44.625)
  line L79 (83.8625, 44.625) -> (69.8625, 44.625)
  line L80 (88.9125, 44.625) -> (88.9125, 58.625)
  line L81 (88.9125, 58.625) -> (102.9125, 58.625)
  line L82 (102.9125, 58.625) -> (102.9125, 44.625)
  line L83 (102.9125, 44.625) -> (88.9125, 44.625)
  line L84 (107.9625, 44.625) -> (107.9625, 58.625)
  line L85 (107.9625, 58.625) -> (121.9625, 58.625)
  line L86 (121.9625, 58.625) -> (121.9625, 44.625)
  line L87 (121.9625, 44.625) -> (107.9625, 44.625)
  line L88 (60.3375, 39.575) -> (74.3375, 39.575)
  line L89 (60.3375, 25.575) -> (60.3375, 39.575)
  line L90 (74.3375, 39.575) -> (74.3375, 25.575)
  line L91 (74.3375, 25.575) -> (60.3375, 25.575)
  line L92 (79.3875, 39.575) -> (93.3875, 39.575)
  line L93 (79.3875, 25.575) -> (79.3875, 39.575)
  line L94 (93.3875, 39.575) -> (93.3875, 25.575)
  line L95 (93.3875, 25.575) -> (79.3875, 25.575)
  line L96 (98.4375, 39.575) -> (112.4375, 39.575)
  line L97 (98.4375, 25.575) -> (98.4375, 39.575)
  line L98 (112.4375, 39.575) -> (112.4375, 25.575)
  line L99 (112.4375, 25.575) -> (98.4375, 25.575)
  circle A3 centre (107.1, 100.15) radius 1.55
  circle A4 centre (101.4156, 3.1) radius 1.55
  point P0 (33.1, 3.1)
  dimension "d385" = 30
  dimension "d386" = 103.25
  dimension "d392" = 14
  dimension "d393" = 14
  dimension "d394" = 6.8
  dimension "d395" = 11.2
  dimension "d396" = 1.5
  dimension "d397" = 4.5
  dimension "d398" = 5.9
  dimension "d400" = 14
  dimension "d401" = 14
  dimension "d402" = 21.7188
  dimension "d443" = 3.1
  dimension "d448" = 3.1
  dimension "d449" = 3.1
  dimension "d450" = 3.1
  dimension "d451" = 3.1
  dimension "d455" = 10.4469
  dimension "d456" = 23.05
  dimension "d457" = 74.5156
  dimension "d458" = 19.05
  dimension "d460" = 9.525
  dimension "d462" = 4.7625
  dimension "d463" = 9.525
  dimension "d464" = 23.05
  dimension "d568" = 80.2
  dimension "d569" = 25.575
  dimension "d570" = 14
  dimension "d571" = 14
  dimension "d572" = 11.2875
  dimension "d573" = 19.05
  dimension "d574" = 19.05
  dimension "d575" = 19.05
  dimension "d576" = 6.525
  dimension "d577" = 16.05
  dimension "d578" = 20.8125
  dimension "d579" = 14
  dimension "d580" = 14
  dimension "d581" = 14
  dimension "d582" = 14
  dimension "d583" = 14
  dimension "d584" = 14
  dimension "d587" = 19.05
  dimension "d588" = 0
  dimension "d591" = 19.05
  dimension "d592" = 0
  dimension "d595" = 19.05
  dimension "d596" = 0
  dimension "d599" = 19.05
  dimension "d600" = 0
  dimension "d601" = 11.2875
  dimension "d602" = 6.525
  dimension "d604" = 3.1
  dimension "d605" = 3.1
  dimension "d606" = 3.1
  dimension "d607" = 3.1
  dimension "d608" = 3.1
  dimension "d609" = 3.1
  dimension "d610" = 3.1
  dimension "d611" = 1.5
  constraint horizontal L11
  constraint vertical L2
  constraint horizontal L2.end origin
  constraint horizontal L35
  constraint vertical L29
  constraint horizontal L18
  constraint vertical L4
  constraint horizontal L21
  constraint vertical L19
  constraint horizontal L13
  constraint vertical L38
  constraint horizontal L6
  constraint horizontal L36
  constraint vertical L34
  constraint horizontal L7
  constraint vertical L16
  constraint collinear L19 L25
  constraint coincident L4.end L20
  constraint collinear L4 L26
  constraint coincident L29.end L6
  constraint collinear L29 L33
  constraint collinear L15 L16
  constraint equal L21 L36
  constraint equal L34 L38
  constraint equal L15 L19
  constraint equal L19 L25
  constraint horizontal L23
  constraint vertical L32
  constraint horizontal L9
  constraint vertical L39
  constraint horizontal A1.centre P0
  constraint vertical A2.centre P0
  constraint perpendicular L43 L44
  constraint perpendicular L45 L46
  constraint perpendicular L46 L47
  constraint perpendicular L10 L49
  constraint perpendicular L11 L50
  constraint perpendicular L44 L51
  constraint perpendicular L45 L51
  constraint perpendicular L47 L48
  constraint perpendicular L43 L50
  constraint horizontal L3
  constraint horizontal L5
  constraint vertical L37
  constraint vertical L31
  constraint vertical L0
  constraint horizontal L28
  constraint vertical L1
  constraint horizontal L8
  constraint horizontal L30
  constraint vertical L14
  constraint vertical L40
  constraint horizontal L27
  constraint horizontal L12
  constraint vertical L22
  constraint horizontal L17
  constraint vertical L41
  constraint horizontal A2.centre A3.centre
  constraint horizontal L4.start L9.start
  constraint equal L6 L42
  constraint horizontal L20
  constraint horizontal L42
  measures "d385" horizontal distance of L2.end origin
  measures "d386" distance of L2.start L2.end
  measures "d392" distance of L26.end L29.start
  measures "d393" distance of L4.start L26.end
  measures "d394" distance of L19.start L21.start
  measures "d395" distance of L13.end L21.start
  measures "d396" distance of L6.end L6.start
  measures "d397" distance of L19.start L6.start
  measures "d398" distance of L6.end L26.end
  measures "d400" distance of L23.start L23.end
  measures "d401" distance of L23.start L9.end
  measures "d402" distance of L4.start L9.start
  measures "d443" diameter of A1
  measures "d448" diameter of A0
  measures "d449" horizontal distance of P0 L2.end
  measures "d450" diameter of A2
  measures "d451" horizontal distance of A2.centre L2.start
  measures "d455" distance of L43.end L43.start
  measures "d456" distance of L43.end L11.end
  measures "d457" distance of L2.end L11.end
  measures "d458" distance of L43.start L44.start
  measures "d460" distance of L44.start L45.start
  measures "d462" distance of L45.end L46.start
  measures "d463" distance of L47.start L48.start
  measures "d464" distance of L48.start L10.start
  measures "d568" distance of L2.start L10.start
  measures "d569" distance of L5.end L11
  measures "d570" distance of L5.end L3.start
  measures "d571" distance of L3.end L3.start
  measures "d572" distance of L5.end L2
  measures "d573" vertical distance of L0.start L5.end
  measures "d574" vertical distance of L14.start L0.start
  measures "d575" vertical distance of L12.end L14.start
  measures "d576" distance of L12.end L2
  measures "d577" distance of L14.start L2
  measures "d578" distance of L0.start L2
  measures "d579" distance of L12.end L17.start
  measures "d580" distance of L17.end L17.start
  measures "d581" distance of L14.end L27.end
  measures "d582" distance of L14.start L14.end
  measures "d583" distance of L1.start L0.end
  measures "d584" distance of L0.start L0.end
  measures "d601" distance of L9.end L2
  measures "d602" distance of L9.end L11
  measures "d604" vertical distance of A2.centre L2.start
  measures "d605" diameter of A3
  measures "d606" horizontal distance of L10.start A3.centre
  measures "d607" vertical distance of P0 L2.end
  measures "d608" diameter of A4
  measures "d609" horizontal distance of L11.end A4.centre
  measures "d610" vertical distance of L11.end A4.centre
  measures "d611" distance of L4.end L24.end